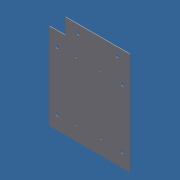
# Autodesk Inventor part: front right plate
Saved by Autodesk Inventor 2012 (Build 160160000, 160)
## iProperties
Created: 2012-03-30
Part Number: front right plate
Material: Aluminum-6061
Document SubType Name: Modeling
Designer: Edward
Density: 2.71 g/cm^3
Mass: 231.465 g
Surface Area: 1093.86 cm^2
Volume: 85.4113 cm^3
Author: Edward
Autodesk Inventor part; units mm, degrees
ref_plane "YZ Plane" through (0, 0, 0) normal (1, 0, 0) x (0, 1, 0)
ref_plane "XZ Plane" through (0, 0, 0) normal (0, 1, 0) x (-1, 0, 0)
ref_plane "XY Plane" through (0, 0, 0) normal (0, 0, 1) x (1, 0, 0)
sketch "Sketch1" plane through (0, 0, 0) normal (0, 0, 1) x (1, 0, 0)
  line L0 (0, 0) -> (209.55, 0)
  line L1 (209.55, 0) -> (209.55, 266.7)
  line L2 (209.55, 266.7) -> (0, 266.7)
  line L3 (0, 266.7) -> (0, 0)
  line L4 (0, 0) -> (41.275, 0)
  line L5 (0, 41.275) -> (0, 0)
  line L6 (0, 266.7) -> (41.275, 266.7)
  line L7 (41.275, 266.7) -> (41.275, 225.425)
  line L8 (41.275, 225.425) -> (0, 225.425)
  line L9 (0, 225.425) -> (0, 266.7)
  dimension "d0" = 266.7
  dimension "d1" = 209.55
  dimension "d4" = 41.275
  constraints: 20 end point, 4 parallel, 3 horizontal, 3 perpendicular
  measures "d0" distance of L2.end L0.start
  measures "d1" distance of L0.start L0.end
  measures "d4" distance of L6.end L7.end
extrude "Extrusion1" add sketch "Sketch1" along normal blind 1.5875 contours L3 L8 L7 L2 L1 L0
sketch "Sketch2" plane through (0, 0, 1.5875) normal (0, 0, 1) x (1, 0, 0)
  line L0 (209.55, 0) -> (0, 0)
  line L1 (209.55, 266.7) -> (209.55, 0)
  line L2 (41.275, 266.7) -> (209.55, 266.7)
  line L3 (20, 188.9125) -> (20, 36.5125)
  line L4 (189.55, 188.9125) -> (189.55, 36.5125)
  line L5 (74.6125, 246.7) -> (176.2125, 246.7)
  line L6 (41.275, 266.7) -> (41.275, 225.425) projected
  line L7 (41.275, 266.7) -> (209.55, 266.7) projected
  line L8 (0, 0) -> (0, 225.425)
  line L9 (0, 225.425) -> (41.275, 225.425)
  point P0 (41.275, 0)
  point P1 (189.55, 112.7125)
  point P2 (125.4125, 246.7)
  point P3 (125.4125, 266.7)
  point P4 (20, 112.7125)
  point P5 (0, 112.7125)
  dimension "d6" = 20
  dimension "d8" = 20
  dimension "d9" = 152.4
  dimension "d10" = 152.4
  dimension "d11" = 101.6
  dimension "d19" = 20
  constraints: 16 end point, 5 midpoint, 3 horizontal alignment, 3 perpendicular, 3 vertical alignment, 1 parallel
  measures "d6" distance from line of L1 L4.start
  measures "d8" distance from line of L2 L5.start
  measures "d9" distance of L3.start L3.end
  measures "d10" distance of L4.start L4.end
  measures "d11" distance of L5.start L5.end
  measures "d19" distance between parallel lines of L8 L3
hole "Hole1" at (20, 188.9125, 1.5875) at (20, 36.5125, 1.5875) at (74.6125, 246.7, 1.5875) at (176.2125, 246.7, 1.5875) at (189.55, 188.9125, 1.5875) at (189.55, 36.5125, 1.5875) direction (0, 0, -1) diameter 8.9916 end through all clearance for "Flat Head Machine Screw" size "M8" standard "Ansi Metric M Profile"
sketch "Sketch3" plane through (0, 0, 1.5875) normal (0, 0, 1) x (1, 0, 0)
  line L0 (0, 0) -> (0, 225.425) projected
  line L1 (41.275, 266.7) -> (209.55, 266.7) projected
  line L2 (69.85, 190.5) -> (133.35, 190.5)
  line L3 (133.35, 190.5) -> (133.35, 31.75)
  line L4 (133.35, 31.75) -> (69.85, 31.75)
  line L5 (69.85, 31.75) -> (69.85, 190.5)
  dimension "d20" = 69.85
  dimension "d21" = 63.5
  dimension "d22" = 158.75
  dimension "d23" = 76.2
  constraints: 8 end point, 2 coincident, 2 parallel, 1 horizontal, 1 perpendicular
  measures "d20" distance between parallel lines of L0 L5
  measures "d21" distance between parallel lines of L3 L5
  measures "d22" distance of L4.end L2.start
  measures "d23" distance between parallel lines of L1 L2
hole "Hole2" at (69.85, 190.5, 1.5875) at (133.35, 190.5, 1.5875) at (69.85, 31.75, 1.5875) at (133.35, 31.75, 1.5875) direction (0, 0, -1) diameter 4.4958 end through all clearance for "Flat Head Machine Screw (82)" size "#8" standard "Ansi Unified Screw Threads"
body "Solid1"
